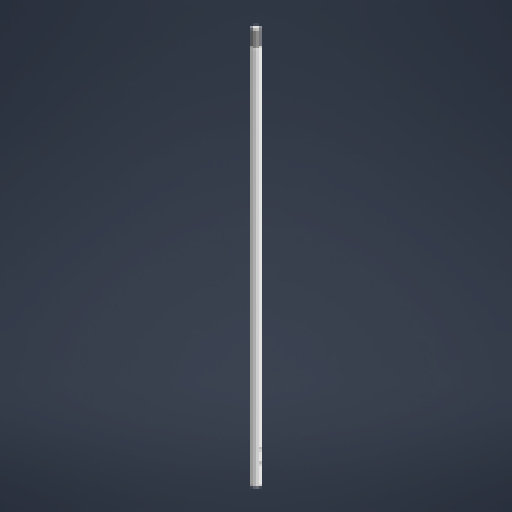
# Autodesk Inventor part: Halterung_Stange
Saved by Autodesk Inventor 2027 (Build 310192060, 192F)
## iProperties
Created: 2026-07-21
Part Number: Halterung_Stange
Material: Generic
Document SubType Name: Modeling
Designer: kw
Density: 1 g/cm^3
Appearance: Default
Author: kw
Autodesk Inventor part; units mm, degrees
ref_plane "XZ Plane" through (0, 0, 0) normal (0, 1, 0) x (-1, 0, 0)
ref_plane "XY Plane" through (0, 0, 0) normal (0, 0, 1) x (1, 0, 0)
sketch "Sketch1" plane through (0, 0, 0) normal (0, 1, 0) x (-1, 0, 0)
  circle A0 centre (0, 0) radius 5
  dimension "d0" = 10
  constraints: 2 coincident, 1 centre point
  measures "d0" diameter of A0
extrude "Extrusion1" add sketch "Sketch1" along normal blind 450
hole "Hole1" at (0, 0, 0) direction (0, 1, 0) diameter 6 depth 15 tip angle 118
thread "Thread1" size "M6x1" class "6H" standard "ISO Metric profile" length 13
ref_plane "Work Plane1" through (-5, 0, 0) normal (1, 0, 0) x (0, 1, 0)
sketch "Sketch2" plane through (-5, 0, 0) normal (1, 0, 0) x (0, 1, 0)
  line L0 (0, 0) -> (14, 0)
  dimension "d12" = 14
  constraints: 2 end point, 1 coincident, 1 horizontal
  measures "d12" distance of L0.start L0.end
hole "Hole2" at (-5, 14, 0) direction (1, 0, 0) diameter 1.5 depth 4
sketch "Sketch3" plane through (-5, 0, 0) normal (1, 0, 0) x (0, 1, 0)
  line L0 (0, 0) -> (25, 0)
  line L1 (0, 0) -> (40, 0)
  dimension "d20" = 25
  dimension "d22" = 40
  constraints: 4 end point, 2 coincident, 1 horizontal
  measures "d20" distance of L0.start L0.end
  measures "d22" distance of L0.start L1.end
hole "Hole3" at (-5, 40, 0) at (-5, 25, 0) direction (1, 0, 0) diameter 3 end through all
thread "Thread2" size "M3x0.5" class "6H" standard "ISO Metric profile" length 13
thread "Thread3" size "M3x0.5" class "6H" standard "ISO Metric profile" length 13
sketch "Sketch4" plane through (0, 450, 0) normal (0, 1, 0) x (1, 0, 0)
  circle A0 centre (0, 0) radius 5 projected
  circle A1 centre (0, 0) radius 4
  dimension "d38" = 8
  constraints: 1 centre point, 1 coincident
  measures "d38" diameter of A1
extrude "Extrusion2" add sketch "Sketch4" along normal blind 40 contours A1
thread "Thread4" size "M8x1.25" class "6g" standard "ISO Metric profile" length 39
chamfer "Chamfer1" distance 1 angle 45 1 edges at (-4, 450, 0)
body "Solid1"
